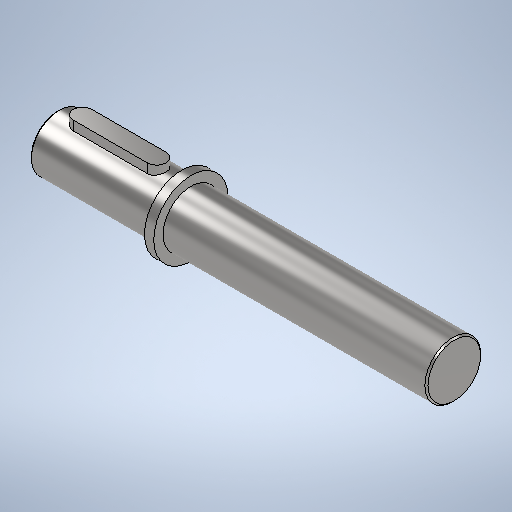
# Autodesk Inventor part: motor_shaft
Saved by Autodesk Inventor 2025.3 (Build 293356030, 356C)
## iProperties
Created: 2025-08-25
Part Number: motor_shaft
Material: 스테인리스스틸
Document SubType Name: Modeling
Designer: MSI
Density: 7.58154 g/cm^3
Appearance: 반연마
Mass: 252 g
Surface Area: 86.3174 cm^2
Volume: 33.2386 cm^3
Author: MSI
Autodesk Inventor part; units mm, degrees
ref_plane "YZ Plane" through (0, 0, 0) normal (1, 0, 0) x (0, 1, 0)
ref_plane "XY Plane" through (0, 0, 0) normal (0, 0, 1) x (1, 0, 0)
sketch "스케치1" plane through (0, 0, 0) normal (1, 0, 0) x (0, 1, 0)
  circle A0 centre (0, 0) radius 9
  dimension "d0" = 18
  constraints: 1 centre point, 1 coincident
  measures "d0" diameter of A0
extrude "돌출1" add sketch "스케치1" along normal blind 40
sketch "스케치2" plane through (40, 0, 0) normal (1, 0, 0) x (0, 0, -1)
  circle A0 centre (0, 0) radius 12
  dimension "d3" = 24
  constraints: 1 centre point, 1 coincident
  measures "d3" diameter of A0
extrude "돌출2" add sketch "스케치2" along normal blind 3
sketch "스케치3" plane through (43, 0, 0) normal (1, 0, 0) x (0, 0, -1)
  circle A0 centre (0, 0) radius 9
  dimension "d6" = 18
  constraints: 1 centre point, 1 coincident
  measures "d6" diameter of A0
extrude "돌출3" add sketch "스케치3" along normal blind 85
ref_plane "작업 평면1" through (0, 9, 0) normal (0, 1, 0) x (-1, 0, 0)
sketch "스케치4" plane through (0, 9, 0) normal (0, 1, 0) x (-1, 0, 0)
  line L0 (-8, 0) -> (-32, 0) construction
  line L1 (-8, 3) -> (-32, 3)
  line L2 (-32, -3) -> (-8, -3)
  arc A0 (-8, -3) -> (-8, 3) centre (-8, 0) ccw
  arc A1 (-32, 3) -> (-32, -3) centre (-32, 0) ccw
  line L3 (0, 9) -> (0, -9) projected
  point P0 (0, 0)
  point P1 (-20, 0)
  point P2 (-5, 0)
  point P3 (-35, 0)
  point P4 (0, 0)
  dimension "d9" = 5
  dimension "d10" = 35
  dimension "d11" = 6
  constraints: 8 end point, 6 point on circle, 4 tangent, 2 centre point, 2 midpoint, 1 horizontal, 1 horizontal alignment, 1 parallel
  measures "d9" distance from line of point (-5, 0) L3
  measures "d10" distance from line of point (-35, 0) L3
  measures "d11" distance between parallel lines of L1 L2
extrude "돌출4" add sketch "스케치4" along normal blind 2.5 and the other way blind 3.5
chamfer "모따기1" distance 0.5 angle 45 2 edges at (128, 0, 9) (0, -9, 0)
sketch "스케치5" plane through (0, 0, 0) normal (-1, 0, 0) x (0, 0, 1)
  circle A0 centre (0, 0) radius 8.5 projected
  constraints: 1 coincident
hole "구멍1" at (0, 0, 0) direction (1, 0, 0) diameter 4.917 depth 18 tip angle 118 thread size "M6x1" class "6H" standard "ISO Metric profile"
chamfer "모따기2" distance 2 angle 30 1 edges at (0, 0, -2.4585) measured on face at (0.5, 0, -2.4585)
